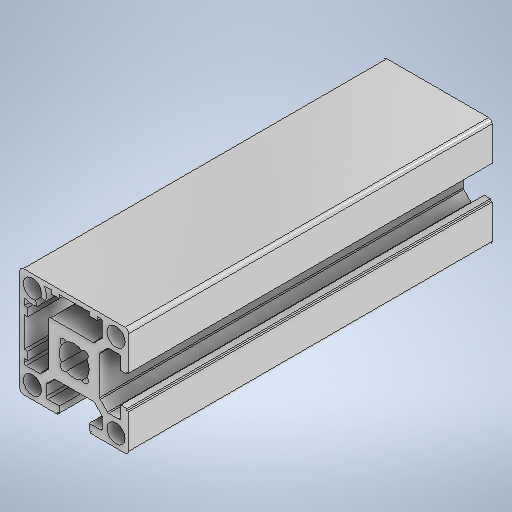
# Autodesk Inventor part: Perfil 30×30 2 rasgos adjacentes
Saved by Autodesk Inventor 2026 (Build 300175000, 175)
## iProperties
Created: 2025-04-05
Part Number: Perfil 30×30 2 rasgos adjacentes
Material: Aluminum 6061
Document SubType Name: Modeling
Designer: Tony Dias
Density: 2.7 g/cm^3
Appearance: Aluminum - Polished
Author: Tony Dias
Autodesk Inventor part; units mm, degrees
sketch "Sketch1" plane through (0, 0, 0) normal (0, 0, 1) x (1, 0, 0)
  circle A0 centre (0, 0) radius 4.1 construction
  line L0 (-15, 15) -> (0, 0) construction
  line L1 (-15, -15) -> (0, 0) construction
  line L2 (-15, 15) -> (0, 15)
  circle A1 centre (-11.5, 11.5) radius 2.5 construction
  line L3 (-15, 15) -> (-15, -15)
  circle A2 centre (-11.5, -11.5) radius 2.5
  line L4 (0, 0) -> (0, -15) construction
  line L5 (0, 0) -> (15, -15) construction
  circle A3 centre (11.5, -11.5) radius 2.5
  circle A4 centre (-2.8991, 2.8991) radius 1 construction
  circle A5 centre (-2.8991, -2.8991) radius 1 construction
  circle A6 centre (2.8991, -2.8991) radius 1 construction
  circle A7 centre (2.8991, 2.8991) radius 1 construction
  line L6 (-7, 7) -> (-7, -7) construction
  arc A8 (-3.5147, 2.1111) -> (-3.5147, -2.1111) centre (0, 0) ccw
  arc A9 (-3.5147, -2.1111) -> (-2.1111, -3.5147) centre (-2.8991, -2.8991) ccw
  arc A10 (-2.1111, -3.5147) -> (2.1111, -3.5147) centre (0, 0) ccw
  arc A11 (2.1111, -3.5147) -> (3.6062, -3.6062) centre (2.8991, -2.8991) ccw
  line L7 (15, -15) -> (-15, 15) construction
  line L8 (-4.1, -12.8) -> (-4.1, -15) construction
  line L9 (-7.75, -12.8) -> (-4.1, -12.8)
  line L10 (-7.75, -9.3056) -> (-7.75, -12.8)
  line L11 (-7, -7) -> (7, -7) construction
  line L12 (-5.4444, -7) -> (-7.75, -9.3056)
  line L13 (-7, -5.4444) -> (-9.3056, -7.75)
  line L14 (-13.75, -7.75) -> (-9.3056, -7.75)
  line L15 (5.4444, -7) -> (7.75, -9.3056)
  line L16 (7.75, -9.3056) -> (7.75, -12.8)
  line L17 (4.1, -12.8) -> (7.75, -12.8)
  line L18 (4.1, -12.8) -> (4.1, -15) construction
  line L19 (4.1, -15) -> (15, -15) construction
  line L20 (-5.4444, -7) -> (5.4444, -7)
  line L21 (-4.1, -15) -> (-4.6, -15) construction
  line L22 (-4.6, -15) -> (-4.6, -14.5)
  line L23 (-4.6, -14.5) -> (-4.1, -14.5)
  line L24 (-4.1, -14.5) -> (-4.1, -15) construction
  line L25 (-4.1, -12.8) -> (-4.1, -14.5)
  line L26 (-15, -15) -> (-4.6, -15)
  line L27 (4.1, -15) -> (4.6, -15) construction
  line L28 (4.6, -15) -> (4.6, -14.5)
  line L29 (4.6, -14.5) -> (4.1, -14.5)
  line L30 (4.1, -14.5) -> (4.1, -15) construction
  line L31 (4.1, -12.8) -> (4.1, -14.5)
  arc A12 (-3.6062, 3.6062) -> (-3.5147, 2.1111) centre (-2.8991, 2.8991) ccw
  line L32 (4.6, -15) -> (15, -15)
  line L33 (-13.75, -4.1) -> (-13.75, -7.75) construction
  line L34 (-12.8, -4.1) -> (-12.8, -6.3)
  line L35 (-12.8, -6.3) -> (-13.75, -6.3)
  line L36 (-13.75, -4.1) -> (-12.8, -4.1)
  line L37 (-13.75, -6.3) -> (-13.75, -7.75)
  line L38 (-13.75, 0) -> (-13.75, -4.1)
  line L39 (0, 0) -> (-15, 0)
  line L40 (-13.75, 4.1) -> (-13.75, 0)
  line L41 (-13.75, 4.1) -> (-12.8, 4.1)
  line L42 (-12.8, 4.1) -> (-12.8, 6.3)
  line L43 (-12.8, 6.3) -> (-13.75, 6.3)
  line L44 (-13.75, 6.3) -> (-13.75, 7.9568)
  line L45 (-7, 7) -> (-7, -5.4444)
  line L46 (-11.5, 11.5) -> (-10.19, 7.9008) construction
  line L47 (-10.6449, 9.1508) -> (-10.19, 7.9008)
  arc A13 (-13.2678, 13.2678) -> (-10.6449, 9.1508) centre (-11.5, 11.5) ccw
  line L48 (-13.2678, 13.2678) -> (-15, 15) construction
  line L49 (-7, 7) -> (-3.6062, 3.6062) construction
  line L50 (15, -15) -> (13.2678, -13.2678)
  arc A14 (-9.1508, 10.6449) -> (-13.2678, 13.2678) centre (-11.5, 11.5) ccw
  line L51 (-11.5, 11.5) -> (-9.1508, 10.6449) construction
  line L52 (-9.1508, 10.6449) -> (-7.9008, 10.19)
  line L53 (-7.9568, 13.75) -> (-6.3, 13.75)
  line L54 (-6.3, 13.75) -> (-6.3, 12.8)
  line L55 (-6.3, 12.8) -> (-4.1, 12.8)
  line L56 (-4.1, 12.8) -> (-4.1, 13.75)
  line L57 (0, 15) -> (15, 15)
  line L58 (0, 21) -> (0, -21) projected
  line L59 (15, 15) -> (15, -15) construction
  line L60 (-4.1, 13.75) -> (0, 13.75)
  line L61 (0, 13.75) -> (4.1, 13.75)
  line L62 (4.1, 13.75) -> (4.1, 12.8)
  line L63 (4.1, 12.8) -> (6.3, 12.8)
  line L64 (6.3, 12.8) -> (6.3, 13.75)
  arc A15 (-13.4554, 8.133) -> (-10.19, 7.9008) centre (-11.5638, 11.6574) ccw
  arc A16 (-13.4554, 8.133) -> (-13.75, 7.9568) centre (-13.55, 7.9568) ccw
  arc A17 (-7.9568, 13.75) -> (-8.133, 13.4554) centre (-7.9568, 13.55) ccw
  arc A18 (-7.9008, 10.19) -> (-8.133, 13.4554) centre (-11.6574, 11.5638) ccw
  line L65 (6.3, 13.75) -> (7.75, 13.75)
  line L66 (7.75, 13.75) -> (7.75, 9.3056)
  circle A19 centre (11.5, 11.5) radius 2.5
  line L67 (15, 15) -> (0, 0) construction
  line L68 (-21, 0) -> (21, 0) projected
  line L69 (-7, 7) -> (5.4444, 7)
  line L70 (7.75, 9.3056) -> (5.4444, 7)
  line L71 (9.3056, 7.75) -> (7, 5.4444)
  line L72 (9.3056, 7.75) -> (12.8, 7.75)
  line L73 (7, -5.4444) -> (9.3056, -7.75)
  line L74 (7, 5.4444) -> (7, -5.4444)
  line L75 (9.3056, -7.75) -> (12.8, -7.75)
  line L76 (12.8, -4.1) -> (12.8, -7.75)
  line L77 (12.8, -4.1) -> (15, -4.1) construction
  line L78 (12.8, 7.75) -> (12.8, 4.1)
  line L79 (12.8, 4.1) -> (15, 4.1) construction
  line L80 (15, 4.1) -> (14.5, 4.1) construction
  line L81 (14.5, 4.1) -> (14.5, 4.6)
  line L82 (14.5, 4.6) -> (15, 4.6)
  line L83 (15, 4.6) -> (15, 4.1) construction
  line L84 (12.8, 4.1) -> (14.5, 4.1)
  line L85 (15, 4.6) -> (15, 15)
  line L86 (15, -4.1) -> (14.5, -4.1) construction
  line L87 (14.5, -4.1) -> (14.5, -4.6)
  line L88 (14.5, -4.6) -> (15, -4.6)
  line L89 (15, -4.6) -> (15, -4.1) construction
  line L90 (12.8, -4.1) -> (14.5, -4.1)
  line L91 (15, -4.6) -> (15, -15)
  arc A20 (-2.1111, 3.5147) -> (-3.6062, 3.6062) centre (-2.8991, 2.8991) ccw
  arc A21 (2.1111, 3.5147) -> (-2.1111, 3.5147) centre (0, 0) ccw
  arc A22 (3.5147, 2.1111) -> (2.1111, 3.5147) centre (2.8991, 2.8991) ccw
  arc A23 (3.5147, -2.1111) -> (3.5147, 2.1111) centre (0, 0) ccw
  arc A24 (3.6062, -3.6062) -> (3.5147, -2.1111) centre (2.8991, -2.8991) ccw
  point P0 (-13.6085, 10.1568)
  point P1 (3.6062, -3.6062)
  point P2 (-4.1, 0)
  point P3 (-7, 0)
  point P4 (-7.5, 15)
  dimension "d0" = 8.2
  dimension "d2" = 15
  dimension "d3" = 15
  dimension "d4" = 15
  dimension "d5" = 15
  dimension "d6" = 5
  dimension "d7" = 11.5
  dimension "d8" = 2
  dimension "d11" = 360
  dimension "d14" = 8
  dimension "d15" = 4.1
  dimension "d16" = 2.2
  dimension "d17" = 1.25
  dimension "d18" = 1.1
  dimension "d21" = 1.25
  dimension "d22" = 0.5
  dimension "d23" = 4.1
  dimension "d24" = 2.2
  dimension "d27" = 25
  dimension "d33" = 2.2
  dimension "d40" = 1.25
  dimension "d44" = 4
  dimension "d45" = 1.25
  dimension "d46" = 0.2
  dimension "d47" = 11.5
  dimension "d48" = 11.5
  constraints: 180 end point, 46 point on circle, 33 equal length, 26 horizontal, 23 centre point, 19 point on line, 18 vertical, 11 parallel, 10 perpendicular, 9 collinear, 8 concentric, 7 coincident, 7 horizontal alignment, 6 vertical alignment, 5 tangent, 4 equal radius, 3 midpoint, 42 other
  measures "d2" horizontal distance of L0.start point (0, 0)
  measures "d3" horizontal distance of point (0, 0) L0.start
  measures "d4" horizontal distance of point (0, 0) L1.start
  measures "d5" horizontal distance of L1.start point (0, 0)
  measures "d6" diameter of A1
  measures "d7" horizontal distance of point (0, 0) L46.start
  measures "d8" diameter of A4
  measures "d14" distance from line of L1.start L6
  measures "d15" horizontal distance of L39.start L8.end
  measures "d16" distance of L8.start L8.end
  measures "d17" distance edge to line of A2 L10
  measures "d18" distance between parallel lines of L12 L1
  measures "d21" distance from line of L3 L14.start
  measures "d22" distance of L21.end L22.end
  measures "d23" vertical distance of point (0, 0) L33.start
  measures "d24" horizontal distance of L1.start L34.end
  measures "d27" angle of L7 L46
  measures "d33" vertical distance of point (-13.608, 10.157) L44.end
  measures "d40" vertical distance of point (-7.5, 15) L53.start
  measures "d44" radius of A15
  measures "d45" vertical distance of L47.start L46.end
  measures "d46" radius of A16
  measures "d47" horizontal distance of A10.centre A19.centre
  measures "d48" horizontal distance of point (0, 0) A19.centre
extrude "Extrusion3" add sketch "Sketch1" along normal mid plane 100 contours L2 L58 L60 L56 L55 L54 L53 A17 A18 L52 A14 A13 L47 A15 A16 L44 L43 L42 L41 L40 L39 L3 | L57 L85 L82 L81 L84 L78 L72 L71 L74 L68 A23 A22 A21 L58 L69 L70 L66 L65 L64 L63 L62 L61 | L39 L38 L36 L34 L35 L37 L14 L13 L45 A8 A9 A10 L58 L20 L12 L10 L9 L25 L23 L22 L26 L3 | L58 A21 A20 A12 A8 L39 L45 L69 | A10 A11 A24 A23 L68 L74 L73 L75 L76 L90 L87 L88 L91 L32 L28 L29 L31 L17 L16 L15 L20 L58
fillet "Fillet1" radius 1 4 edges at (-15, 15, 0) (15, 15, 0) (-15, -15, 0) (15, -15, 0)
fillet "Fillet2" radius 0.5 26 edges at (-13.75, -7.75, 25) (-13.75, -7.75, -25) (7, 5.4444, 0) (9.3056, 7.75, 0) (7.75, 13.75, 25) (7.75, 13.75, -25) (-9.3056, -7.75, 25) (-9.3056, -7.75, -25) (-7, -5.4444, 25) (-7, -5.4444, -25) (12.8, -7.75, 0) (9.3056, -7.75, 0) (-7, 7, 25) (-7, 7, -25) (5.4444, 7, 25) (5.4444, 7, -25) (7.75, 9.3056, 25) (7.75, 9.3056, -25) (7.75, -12.8, 0) (-7.75, -12.8, 0) (-7.75, -9.3056, 0) (-5.4444, -7, 0) (5.4444, -7, 0) (7.75, -9.3056, 0) (7, -5.4444, 0) (12.8, 7.75, 0)
equation "\"d2\" = d3"
equation "\"d4\" = d3"
equation "\"d5\" = d3"
equation "\"d21\" = d17"
equation "\"d24\" = d16"
body "Solid3"
